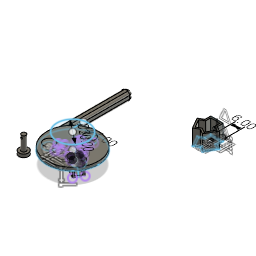
Mini-tri v3 (Autodesk Fusion 360 design; units mm, degrees)
Autodesk Fusion 360 part; units mm, degrees
sketch "Sketch1" plane through (0, 0, 0) normal (0, 1, 0) x (1, 0, 0)
  line L0 (2.4999, 0) -> (2.5, 0)
  line L1 (5, 2.5) -> (5, 53)
  line L2 (3, 55) -> (2, 55)
  line L3 (0, 53) -> (0, 2.5)
  arc A0 (2, 55) -> (0, 53) centre (2, 53) ccw
  arc A1 (5, 53) -> (3, 55) centre (3, 53) ccw
  arc A2 (0, 2.5) -> (2.4999, 0) centre (2.5, 2.5) ccw
  arc A3 (2.5, 0) -> (5, 2.5) centre (2.5, 2.5) ccw
  circle A4 centre (2.5, 2.5) radius 1.5
  line L4 (0, 5) -> (5, 5)
  point P0 (5, 0)
  point P1 (0, 55)
  dimension "d1" = 5
  dimension "d2" = 55
  dimension "d3" = 2
  dimension "d4" = 2
  dimension "d5" = 2.5
  dimension "d6" = 2.5
  dimension "d7" = 3
  constraint vertical L1
  constraint horizontal L2
  constraint vertical L3
  constraint coincident P1 L3
  constraint coincident P1 L2
  constraint tangent L3 A0
  constraint tangent L2 A0
  constraint tangent L1 A1
  constraint tangent L2 A1
  constraint coincident origin L3
  constraint tangent L3 A2
  constraint coincident P0 L1
  constraint coincident P0 L0
  constraint tangent L1 A3
  constraint tangent L0 A3
  constraint concentric A3 A4
  constraint coincident L3 L4.start
  constraint coincident L1 L4.end
  constraint perpendicular L1 L4
  measures "d1" distance of origin P0
  measures "d2" distance of origin P1
  measures "d3" radius of A0
  measures "d4" radius of A1
  measures "d5" radius of A2
  measures "d6" radius of A3
  measures "d7" diameter of A4
extrude "Extrude1" add sketch "Sketch1" along normal blind 5 contours L1 L2 L3 A0 A1 L4 makes body 1
extrude "Extrude2" add sketch "Sketch1" along normal blind 2 contours L1 L3 A2 A3 L4 bodies 1
chamfer "Chamfer1" distance 3 angle 45 1 edges at (2.5, 5, -5) on bodies 1
fillet "Fillet1" radius 1.5 5 edges at (5, 5, -30.5) (4.4142, 5, -54.4142) (2.5, 5, -55) (0.5858, 5, -54.4142) (0, 5, -30.5) on bodies 1
sketch "Sketch2" plane through (5, 0, 0) normal (1, 0, 0) x (0, 0, -1)
  line L0 (53, 3.5) -> (6.5, 3.5)
  line L1 (6.5, 3.5) -> (5, 2)
  line L2 (5, 2) -> (2.5, 2)
  line L3 (2.5, 2) -> (2.5, 0)
  line L4 (2.5, 0) -> (53, 0)
  line L5 (53, 0) -> (53, 3.5)
  line L6 (5, 2) -> (5, 0)
  point P0 (5, 0)
  constraint coincident L1.end L2.start
  constraint coincident P0 L6.end
sketch "Sketch3" plane through (0, 0, 0) normal (-1, 0, 0) x (0, 0, 1)
  line L0 (-6.5, 3.5) -> (-53, 3.5)
  line L1 (-53, 3.5) -> (-53, 0)
  line L2 (-53, 0) -> (-2.5, 0)
  line L3 (-2.5, 0) -> (-2.5, 2)
  line L4 (-2.5, 2) -> (-5, 2)
  line L5 (-5, 2) -> (-6.5, 3.5)
  line L6 (-5, 2) -> (-5, 0)
  line L7 (-5, 0, 0) -> (-5, 0, -5)
  line L8 (-5, 0, -5) -> (-5, 2, -5)
  line L9 (-5, 2, -5) -> (-5, 2, 0)
  point P0 (-5, 0)
  point P1 (-5, 0)
  point P2 (-5, 2)
  constraint coincident P2 L4.end
  constraint coincident P1 P0
sketch "Sketch4" plane through (0, 0, 0) normal (-1, 0, 0) x (0, 0, 1)
ref_plane "WorkPlane1" through (0, 0, -5) normal (0, 0, 1) x (1, 0, 0)
split "Split1" by plane through (0, 0, -5) normal (0, 0, 1) bodies 1 makes body 2 at (3.9981, 1.3333, -2.4252)
fillet "Fillet2" chord length 2 5 edges at (5, 0, -29) (4.4142, 0, -54.4142) (2.5, 0, -55) (0.5858, 0, -54.4142) (0, 0, -29) on bodies 1
fillet "Fillet3" chord length 1 5 faces at (5, 1.3333, -4.1667) (4.3093, 1.3333, -0.7748) (2.5, 0.6667, 0) (2.0268, 1.3333, -0.0452) (0, 1.3333, -4.1667) on bodies 2
sketch "Sketch5" plane through (0, 0, 0) normal (0, 1, 0) x (1, 0, 0)
  line L0 (18.5, 10.5) -> (18.5, 1.7321)
  line L1 (18.5, 1.7321) -> (10.9067, -2.6519)
  line L2 (10.9067, -2.6519) -> (13.9067, -7.8481)
  line L3 (13.9067, -7.8481) -> (21.5, -3.4641)
  line L4 (21.5, -3.4641) -> (29.0933, -7.8481)
  line L5 (29.0933, -7.8481) -> (32.0933, -2.6519)
  line L6 (32.0933, -2.6519) -> (24.5, 1.7321)
  line L7 (24.5, 1.7321) -> (24.5, 10.5)
  line L8 (24.5, 10.5) -> (18.5, 10.5)
  line L9 (14.2728, -6.4821) -> (21.5, -2.3094)
  line L10 (21.5, -2.3094) -> (28.7272, -6.4821)
  line L11 (30.7272, -3.0179) -> (23.5, 1.1547)
  line L12 (23.5, 1.1547) -> (23.5, 9.5)
  line L13 (19.5, 9.5) -> (19.5, 1.1547)
  line L14 (19.5, 1.1547) -> (12.2728, -3.0179)
  line L15 (12.2728, -3.0179) -> (11.4067, -3.5179)
  line L16 (14.2728, -6.4821) -> (13.4067, -6.9821)
  line L17 (28.7272, -6.4821) -> (29.5933, -6.9821)
  line L18 (30.7272, -3.0179) -> (31.5933, -3.5179)
  line L19 (23.5, 9.5) -> (23.5, 10.5)
  line L20 (19.5, 9.5) -> (19.5, 10.5)
  constraint coincident L2 L15.end
  constraint perpendicular L2 L15
  constraint coincident L2 L16.end
  constraint perpendicular L2 L16
  constraint coincident L5 L17.end
  constraint perpendicular L5 L17
  constraint coincident L5 L18.end
  constraint perpendicular L5 L18
  constraint coincident L8 L19.end
  constraint perpendicular L8 L19
  constraint coincident L8 L20.end
  constraint perpendicular L8 L20
extrude "Extrude3" add sketch "Sketch5" along normal blind 8 separate body contours L0 L1 L2 L8 L13 L14 L15 L20 | L5 L6 L7 L8 L11 L12 L18 L19 | L2 L3 L4 L5 L9 L10 L16 L17 makes body 3 at (16.8022, 2.6667, 0.4028) makes body 4 at (23.5, 2.6667, -4.2698) makes body 5 at (24.1978, 2.6667, 3.867)
extrude "Extrude4" add sketch "Sketch5" along normal blind 1 contours L2 L5 L8 L9 L10 L11 L12 L13 L14 L15 L16 L17 L18 L19 L20 bodies 3 4 5
sketch "Sketch6" plane through (3.875, 0, -6.7117) normal (-0.5, 0, 0.866025) x (0.866025, 0, 0.5)
  line L0 (20.3516, 0) -> (29.1195, 0)
  line L1 (29.1195, 0) -> (29.1195, 8)
  line L2 (29.1195, 8) -> (20.3516, 8)
  line L3 (20.3516, 8) -> (20.3516, 0)
  line L4 (20.3516, 8) -> (24.7356, 8)
  line L5 (24.7356, 0) -> (24.7356, 8)
  line L6 (20.3516, 4) -> (29.1195, 4)
  line L7 (24.7356, 4) -> (29.1195, 4)
  constraint coincident L2.end L3.start
  constraint midpoint L2 L4.end
  constraint midpoint L0 L5.start
  constraint midpoint L3 L6.start
  constraint midpoint L1 L6.end
  constraint midpoint L6 L7.start
hole "Hole1" at (25.2966, 4, 5.6561) direction (0.5, 0, -0.866025) diameter 3.1 depth 8 tip angle 118 bodies 3
sketch "Sketch7" plane through (6.875, 0, 11.9078) normal (0.5, 0, 0.866025) x (0.866025, 0, -0.5)
  line L0 (8.1195, 0) -> (16.8875, 0)
  line L1 (16.8875, 0) -> (16.8875, 8)
  line L2 (16.8875, 8) -> (8.1195, 8)
  line L3 (8.1195, 8) -> (8.1195, 0)
  line L4 (18.6222, 8, 1.8079) -> (17.9879, 7.1966, 1.9059)
ref_plane "WorkPlane2" through (17.7034, 4, 5.6561) normal (0.5, 0, 0.866025) x (0.866025, 0, -0.5)
sketch "Sketch8" plane through (17.7034, 4, 5.6561) normal (0.5, 0, 0.866025) x (0.866025, 0, -0.5)
  line L0 (4.384, -4, -6) -> (4.384, 4, -6)
  line L1 (-4.384, -4, -6) -> (-4.384, 4, -6)
  line L2 (4.384, 0, -6) -> (-4.384, 0, -6)
  line L3 (4.384, -4, -6) -> (-4.384, -4, -6)
  line L4 (0, -4, -6) -> (0, 0, -6)
hole "Hole2" at (14.7034, 4, 0.4599) direction (0.5, 0, 0.866025) diameter 3.1 depth 8 tip angle 118 bodies 3
sketch "Sketch9" plane through (18.5, 0, 0) normal (-1, 0, 0) x (0, 0, 1)
  line L0 (-10.5, 0) -> (-1.7321, 0)
  line L1 (-1.7321, 0) -> (-1.7321, 8)
  line L2 (-1.7321, 8) -> (-10.5, 8)
  line L3 (-10.5, 8) -> (-10.5, 0)
  line L4 (-10.5, 4) -> (-1.7321, 4)
  line L5 (-6.116, 0) -> (-6.116, 4)
  constraint midpoint L3 L4.start
  constraint midpoint L1 L4.end
  constraint midpoint L0 L5.start
  constraint midpoint L4 L5.end
hole "Hole3" at (18.5, 4, -6.116) direction (1, 0, 0) diameter 3.1 depth 8 tip angle 118 bodies 3
cylinder "CylinderPrimitive1" add diameter 2.9 height 11 placed x (1, 0, 0) y (0, 0, -1) z (0, 1, 0) at (0, 0, 10) separate body makes body 6
cylinder "CylinderPrimitive2" add diameter 6 height -2 placed x (1, 0, 0) y (0, 0, 1) z (0, -1, 0) at (0, 0, 10) bodies 6
hole "Hole4" at (0, 9.4314, 11.45) direction (0, 0, -1) diameter 1.1 depth 8 tip angle 118 bodies 6
combine "Combine1" operation add target body 2 tool bodies 1
ref_plane "WorkPlane3" through (21.5, 8, 5.0787) normal (0, 1, 0) x (0, 0, 1)
ref_plane "WorkPlane4" through (21.5, 18, 5.0787) normal (0, 1, 0) x (0, 0, 1)
sketch "Sketch12" plane through (21.5, 18, 5.0787) normal (0, 1, 0) x (1, 0, 0)
  circle A0 centre (0, 5) radius 10
  dimension "d46" = 20
  measures "d46" diameter of A0
sketch "Sketch13" plane through (0, 0, 0) normal (0, 1, 0) x (1, 0, 0)
  circle A0 through (23.5, 4.566, 4) (23.5, 6.891, 5.3423) (23.5, 6.891, 2.6577)
  line L0 (22.9058, -0.3067, 1) -> (23.5, 6.116, 4)
  line L1 (29.0933, -7.8481) -> (32.0933, -2.6519)
  line L2 (21.5, -0.0787, 20) -> (30.5933, -5.25, 0)
  line L3 (21.5, -0.0787, 20) -> (21.5, 6.9213, 20)
  dimension "d49" = 7
ref_plane "WorkPlane5" through (21.5, 16, -1.759) normal (0, 1, 0) x (0, 0, 1)
sketch "Sketch14" plane through (21.5, 16, -1.759) normal (0, 1, 0) x (1, 0, 0)
sketch "Sketch15" plane through (21.5, 8, 5.0787) normal (0, 1, 0) x (1, 0, 0)
  line L0 (5.4543, 5.3938) -> (8.139, 3.8438)
  line L1 (3, 12.7448) -> (3, 9.6448)
  line L2 (-2, 12.7448) -> (-2, 9.6448)
  line L3 (2, 12.7448) -> (2, 9.6448)
  line L4 (-3, 9.6448) -> (-3, 12.7448)
  line L5 (3, 6.8108) -> (3, 15.5787)
  line L6 (5.139, -1.3524) -> (2.4543, 0.1976)
  line L7 (7.639, 2.9778) -> (4.9543, 4.5278)
  line L8 (2.9543, 1.0637) -> (5.639, -0.4863)
  line L9 (-2.4543, 0.1976) -> (-5.139, -1.3524)
  line L10 (-5.639, -0.4863) -> (-2.9543, 1.0637)
  line L11 (-8.139, 3.8438) -> (-5.4543, 5.3938)
  line L12 (-4.9543, 4.5278) -> (-7.639, 2.9778)
  line L13 (4.9543, 4.5278) -> (7.639, 2.9778) construction
  circle A0 through (7.639, 2.9778, -4) (5.6255, 4.1403, -2.6577) (5.6255, 4.1403, -5.3423)
  line L14 (4.9543, 4.5278, 0) -> (6.2966, 3.7528, -4)
  line L15 (2.9543, 1.0637) -> (4.2966, 0.2887)
  line L16 (2.9543, 1.0637) -> (5.639, -0.4863) construction
  line L17 (2.9543, 1.0637) -> (4.2966, 0.2887)
  line L18 (5.639, -0.4863) -> (4.2966, 0.2887)
  line L19 (5.639, -0.4863) -> (2.9543, 1.0637)
  line L20 (7.639, 2.9778) -> (6.2966, 3.7528)
  line L21 (6.2966, 3.7528) -> (4.9543, 4.5278)
  line L22 (6.2966, 3.7528) -> (4.2966, 0.2887)
  line L23 (5.2966, 2.0207) -> (7.0287, 1.0207)
  line L24 (0, 5) -> (0, 16)
  circle A1 centre (0, 16) radius 3.5
  circle A2 centre (0, 5) radius 16.5
  circle A3 centre (-9.5263, -0.5) radius 3.5
  circle A4 centre (9.5263, -0.5) radius 3.5
  point P0 (-3, 11.1948)
  dimension "d54" = 2
  dimension "d55" = 7
  dimension "d58" = 360
  constraint coincident L7.end L13.start
  constraint coincident L7.start L13.end
  constraint coincident L20.end L21.start
  constraint coincident L8.start L15.start
  constraint midpoint L8 L15.end
  constraint coincident L8.end L16.end
  constraint midpoint L13 L20.end
  constraint perpendicular L22 L23
  constraint parallel L2 L24
  constraint coincident L24.end A1.centre
  measures "d54" distance of L23.start L23.end
  measures "d55" diameter of A1
extrude "Extrude6" add sketch "Sketch15" along normal blind 2 separate body makes body 7
extrude "Extrude7" add sketch "Sketch15" along normal blind 2 separate body contours A1 | A2 | A3 | A4 makes body 8
copy_body "CopyPasteBodies1" bodies 3 makes body 9
sketch "Sketch16" plane through (0, 0, 0) normal (0, 1, 0) x (1, 0, 0)
  line L0 (50, 60) -> (56, 60)
  line L1 (56, 60) -> (56, 56.7321)
  line L2 (50, 56.7321) -> (50, 60)
  line L3 (53, 51.5359) -> (50.1699, 49.9019)
  line L4 (50.1699, 49.9019) -> (47.1699, 55.0981)
  line L5 (47.1699, 55.0981) -> (50, 56.7321)
  line L6 (56, 56.7321) -> (58.8301, 55.0981)
  line L7 (58.8301, 55.0981) -> (55.8301, 49.9019)
  line L8 (55.8301, 49.9019) -> (53, 51.5359)
  line L9 (56.1962, 48.5359) -> (53, 50.3812)
  line L10 (53, 50.3812) -> (49.8038, 48.5359)
  line L11 (49.8038, 48.5359) -> (45.8038, 55.4641)
  line L12 (45.8038, 55.4641) -> (49, 57.3094)
  line L13 (49, 57.3094) -> (49, 61)
  line L14 (49, 61) -> (57, 61)
  line L15 (57, 61) -> (57, 57.3094)
  line L16 (57, 57.3094) -> (60.1962, 55.4641)
  line L17 (60.1962, 55.4641) -> (56.1962, 48.5359)
  dimension "d63" = 6
  dimension "d67" = -1
  constraint horizontal L0
  constraint vertical L1
  constraint vertical L2
  measures "d63" distance of L0.start L0.end
extrude "Extrude8" add sketch "Sketch16" along normal blind 2 separate body contours L0 L1 L2 L3 L4 L5 L6 L7 L8 makes body 10
extrude "Extrude9" add sketch "Sketch16" along normal blind 10 bodies 10
sketch "Sketch17" plane through (0, 0, -61) normal (0, 0, -1) x (-1, 0, 0)
  line L0 (-57, 0) -> (-49, 0)
  line L1 (-49, 0) -> (-49, 10)
  line L2 (-49, 10) -> (-57, 10)
  line L3 (-57, 10) -> (-57, 0)
  line L4 (-53, 0) -> (-53, 10)
  line L5 (-53, 10) -> (-53, 6)
  constraint midpoint L0 L4.start
  constraint midpoint L2 L4.end
  constraint coincident L4 L5.end
  constraint perpendicular L2 L5
ref_plane "WorkPlane7" through (55, 5, -61) normal (0, 0, -1) x (-1, 0, 0)
sketch "Sketch18" plane through (58.3695, 0, -33.6997) normal (-0.866025, 0, 0.5) x (0.5, 0, 0.866025)
  line L0 (-25.1314, 0) -> (-17.1314, 0)
  line L1 (-17.1314, 0) -> (-17.1314, 10)
  line L2 (-17.1314, 10) -> (-25.1314, 10)
  line L3 (-25.1314, 10) -> (-25.1314, 0)
  line L4 (-21.1314, 10) -> (-21.1314, 0)
  line L5 (-21.1314, 5) -> (-21.1314, 0)
  circle A0 centre (-21.1314, 5) radius 1.55
  line L6 (-15.9352, 5, -9) -> (-21.1314, 10, 0)
  line L7 (-21.1314, 0) -> (-21.1314, 10)
  line L8 (-21.1314, 10) -> (-10.5, 6.5)
  line L9 (-10.5, 6.5, 0) -> (-15.9352, 5, -9)
  line L10 (-13.9352, 10, -5.5359) -> (-17.9352, 10, -12.4641)
  line L11 (-15.9352, 10, -9) -> (-15.9352, 5, -9)
  line L12 (-15.9352, 10, -9) -> (-28.3275, 0, -5.5359)
  point P0 (-28.3275, 0)
  dimension "d72" = 3.1
  constraint midpoint L2 L4.start
  constraint midpoint L0 L4.end
  constraint midpoint L4 L5.start
  constraint coincident L5.start A0.centre
  measures "d72" diameter of A0
ref_plane "WorkPlane6" through (58.1962, 5, -52) normal (0.866025, 0, 0.5) x (0.5, 0, -0.866025)
sketch "Sketch19" plane through (58.1962, 5, -52) normal (0.866025, 0, 0.5) x (0.5, 0, -0.866025)
  line L0 (0, 5) -> (0, 0)
  line L1 (0, 0) -> (0, 5)
  circle A0 centre (0, 0) radius 1.55
  line L2 (7.1962, 5, -5.5359) -> (3.1962, 5, -12.4641)
  line L3 (5.1962, 5, -9) -> (5.1962, -5, -9)
  line L4 (5.1962, -5, -9) -> (5.1962, 0, -9)
  line L5 (5.1962, 5, -9) -> (5.1962, 0, -9)
  point P0 (0, 5)
  point P1 (5.1962, -5)
  point P2 (5.1962, 5)
  dimension "d74" = 3.1
  constraint coincident P0 L0.start
  constraint coincident L0.end L1.start
  measures "d74" diameter of A0
sketch "Sketch20" plane through (0, 0, -61) normal (0, 0, -1) x (1, 0, 0)
  line L0 (53, -10) -> (53, -5)
  circle A0 centre (53, -5) radius 1.55
  point P0 (53, -10)
  point P1 (53, -5)
  dimension "d76" = 3.1
  constraint coincident P0 L0.start
  constraint coincident P1 L0.end
  measures "d76" diameter of A0
extrude "Extrude10" cut sketch "Sketch20" against normal blind 5 bodies 10
extrude "Extrude11" cut sketch "Sketch18" against normal blind 3 contours L4 L5 A0 L7 | L4 L5 A0 L7 bodies 10
extrude "Extrude12" cut sketch "Sketch19" against normal blind 3 bodies 10
sketch "Sketch21" plane through (0, 2, 0) normal (0, 1, 0) x (-1, 0, 0)
  line L0 (-55.8301, -49.9019) -> (-58.8301, -55.0981)
  line L1 (-58.8301, -55.0981) -> (-56, -56.7321)
  line L2 (-56, -56.7321) -> (-56, -60)
  line L3 (-56, -60) -> (-50, -60)
  line L4 (-50, -60) -> (-50, -56.7321)
  line L5 (-50, -56.7321) -> (-47.1699, -55.0981)
  line L6 (-47.1699, -55.0981) -> (-50.1699, -49.9019)
  line L7 (-50.1699, -49.9019) -> (-53, -51.5359)
  line L8 (-53, -51.5359) -> (-55.8301, -49.9019)
  line L9 (-53, -60) -> (-53, -55)
  circle A0 centre (-53, -55) radius 2.75
  dimension "d83" = 5.5
  constraint midpoint L3 L9.start
  constraint perpendicular L3 L9
  constraint coincident L9.end A0.centre
  measures "d83" diameter of A0
extrude "Extrude13" cut sketch "Sketch21" against normal blind 3 contours A0 bodies 10
